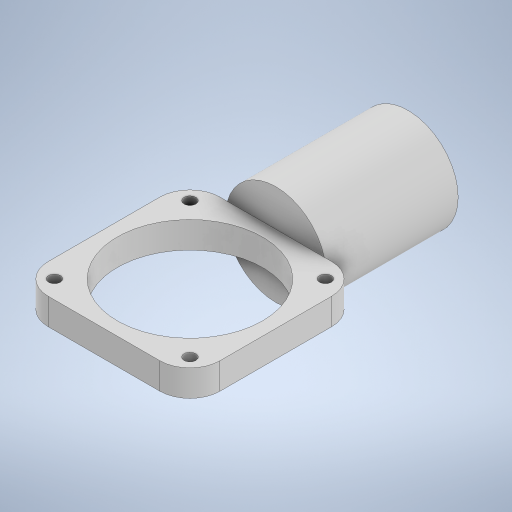
# Autodesk Inventor part: FrontPlateV2
Saved by Autodesk Inventor 2024 (Build 280153000, 153)
## iProperties
Created: 2024-02-08
Part Number: FrontPlateV2
Material: Generic
Document SubType Name: Modeling
Designer: yusuf
Density: 1 g/cm^3
Appearance: Default
Author: yusuf
Autodesk Inventor part; units mm, degrees
ref_plane "YZ Plane" through (0, 0, 0) normal (1, 0, 0) x (0, 1, 0)
ref_plane "XZ Plane" through (0, 0, 0) normal (0, 1, 0) x (-1, 0, 0)
ref_plane "XY Plane" through (0, 0, 0) normal (0, 0, 1) x (1, 0, 0)
sketch "Sketch1" plane through (0, 0, 0) normal (0, 0, 1) x (1, 0, 0)
  circle A0 centre (0, 0) radius 38
  dimension "d0" = 76
  constraints: 1 centre point, 1 coincident
  measures "d0" diameter of A0
extrude "Extrusion1" add sketch "Sketch1" along normal blind 100
sketch "Sketch2" plane through (0, 0, 0) normal (0, 0, -1) x (-1, 0, 0)
  circle A0 centre (0, 0) radius 8.75
  line L0 (0, 8.75) -> (0, 11.75)
  line L1 (0, 11.75) -> (4, 11.75)
  line L2 (4, 11.75) -> (-4, 11.75)
  line L3 (-4, 11.75) -> (-4, 7.7822)
  line L4 (4, 11.75) -> (4, 7.7822)
  dimension "d3" = 17.5
  dimension "d5" = 3
  dimension "d6" = 4
  dimension "d7" = 8
  dimension "d8" = 3.9678
  dimension "d9" = 3.9678
  constraints: 10 end point, 3 point on circle, 2 vertical, 1 centre point, 1 coincident, 1 horizontal, 1 point on line
  measures "d3" diameter of A0
  measures "d5" distance of L0.start L0.end
  measures "d6" distance of L0.end L1.end
  measures "d7" distance of L1.end L2.end
  measures "d8" distance of L2.end L3.end
  measures "d9" distance of L1.end L4.end
extrude "Extrusion2" cut sketch "Sketch2" against normal blind 90
fillet "Fillet1" radius 0.5 4 edges at (4, 9.7661, 0) (0, 11.75, 0) (-4, 9.7661, 0) (0, -8.75, 0)
fillet "Fillet2" radius 0.5 4 edges at (-4, 7.7822, 45.25) (-4.1498, 7.8731, 0.1431) (4, 7.7822, 45.25) (4.1498, 7.8731, 0.1431)
sketch "Sketch5" plane through (0, 0, 100) normal (0, 0, 1) x (1, 0, 0)
  line L0 (-65, -10) -> (65, -10)
  line L1 (65, -10) -> (65, 10)
  line L2 (65, 10) -> (-65, 10)
  line L3 (-65, 10) -> (-65, -10)
  line L4 (-65, -10) -> (65, 10) construction
  line L5 (65, -10) -> (-65, 10) construction
  point P0 (0, 0)
  dimension "d32" = 130
  dimension "d33" = 20
  constraints: 12 end point, 2 midpoint, 2 parallel, 1 horizontal, 1 perpendicular
  measures "d32" distance of L1.end L2.end
  measures "d33" distance of L0.end L1.end
extrude "Extrusion5" add sketch "Sketch5" along normal blind 130
fillet "Fillet6" radius 22.751 4 edges at (-65, 0, 230) (65, 0, 230) (65, 0, 100) (-65, 0, 100)
sketch "Sketch6" plane through (-36.6606, 10, 100) normal (0, 1, 0) x (1, 0, 0)
  circle A0 centre (36.6606, -65) radius 55
  line L0 (-28.3394, 0) -> (-28.3394, -130) projected
  line L1 (101.6606, -130) -> (-28.3394, -130) projected
  point P0 (36.6606, 100)
  point P1 (-33.3394, -33)
  dimension "d39" = 110
  dimension "d40" = 65
  dimension "d41" = 65
  constraints: 1 centre point, 1 other
  measures "d39" diameter of A0
  measures "d41" distance from line of A0.centre L1
extrude "Extrusion6" cut sketch "Sketch6" against normal blind 20
sketch "Sketch7" plane through (-36.6606, 10, 100) normal (0, 1, 0) x (1, 0, 0)
  line L0 (-28.3394, -22.751) -> (-28.3394, -107.249) projected
  arc A0 (-28.3394, -107.249) -> (-5.5884, -130) centre (-5.5884, -107.249) ccw projected
  circle A1 centre (-14.6044, -116.265) radius 4.5
  circle A2 centre (-14.6044, -13.735) radius 4.5
  circle A3 centre (87.9256, -13.735) radius 4.5
  circle A4 centre (87.9256, -116.265) radius 4.5
  line L1 (78.9096, -130) -> (-5.5884, -130) projected
  line L2 (101.6606, -22.751) -> (101.6606, -107.249) projected
  line L3 (0, 0) -> (73.3212, 0) projected
  line L4 (0, 0) -> (-5.5884, 0) projected
  point P0 (36.6606, 100)
  dimension "d45" = 9
  dimension "d46" = 13.735
  dimension "d47" = 13.735
  dimension "d50" = 9
  dimension "d51" = 13.735
  dimension "d52" = 13.735
  dimension "d53" = 9
  dimension "d54" = 13.735
  dimension "d55" = 13.735
  dimension "d56" = 9
  dimension "d57" = 13.735
  dimension "d58" = 13.735
  constraints: 4 centre point
  measures "d45" diameter of A1
  measures "d46" horizontal distance of L0.end A1.centre
  measures "d47" vertical distance of L1.end A1.centre
  measures "d50" diameter of A4
  measures "d51" distance from line of L1 A4.centre
  measures "d52" distance from line of L2 A4.centre
  measures "d53" diameter of A3
  measures "d54" distance from line of L2 A3.centre
  measures "d55" distance from line of L3 A3.centre
  measures "d56" diameter of A2
  measures "d57" distance from line of L0 A2.centre
  measures "d58" distance from line of L4 A2.centre
extrude "Extrusion7" cut sketch "Sketch7" against normal blind 20
equation "\"d47\" = d46"
equation "\"d52\" = d51"
equation "\"d55\" = d54"
equation "\"d57\" = d46"
equation "\"d58\" = d57"
body "Solid1"
